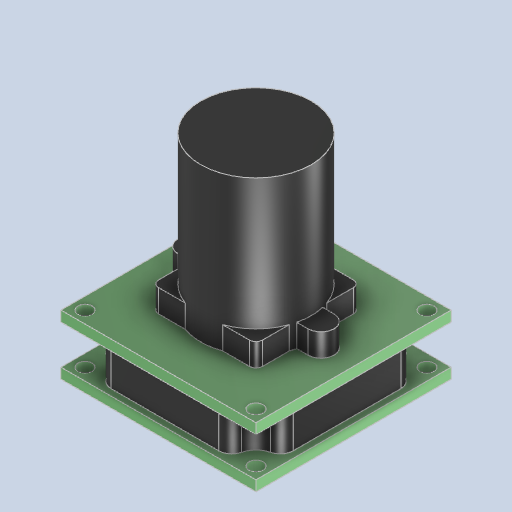
# Autodesk Inventor part: e-CAM50_CUNX
Saved by Autodesk Inventor 2022.3 (Build 263350000, 350)
## iProperties
Created: 2023-04-07
Part Number: e-CAM50_CUNX
Material: Generic
Document SubType Name: Modeling
Designer: Masato Kubotera
Density: 1 g/cm^3
Appearance: 光沢 - 黒
Catalog Web Link: https://www.e-consystems.com/nvidia-cameras/jetson-nx-cameras/5mp-mipi-camera-board-jp.asp
Description: ReadyMade
Author: Masato Kubotera
Autodesk Inventor part; units mm, degrees
ref_plane "YZ Plane" through (0, 0, 0) normal (1, 0, 0) x (0, 1, 0)
ref_plane "XZ Plane" through (0, 0, 0) normal (0, 1, 0) x (-1, 0, 0)
sketch "スケッチ1" plane through (0, 0, 0) normal (0, 0, 1) x (1, 0, 0)
  line L0 (-15, -15) -> (15, -15)
  line L1 (15, -15) -> (15, 15)
  line L2 (15, 15) -> (-15, 15)
  line L3 (-15, 15) -> (-15, -15)
  line L4 (-15, -15) -> (15, 15) construction
  line L5 (15, -15) -> (-15, 15) construction
  line L6 (-15, 0) -> (15, 0) construction
  line L7 (0, 15) -> (0, -15) construction
  line L8 (-13.14, 13.14) -> (13.14, 13.14) construction
  line L9 (13.14, 13.14) -> (13.14, -13.14) construction
  line L10 (13.14, -13.14) -> (-13.14, -13.14) construction
  line L11 (-13.14, -13.14) -> (-13.14, 13.14) construction
  line L12 (-13.14, 13.14) -> (13.14, -13.14) construction
  line L13 (13.14, 13.14) -> (-13.14, -13.14) construction
  circle A0 centre (0, 0) radius 8.5
  line L14 (-7, 8) -> (7, 8)
  line L15 (8, 7) -> (8, -7)
  line L16 (7, -8) -> (-7, -8)
  line L17 (-8, -7) -> (-8, 7)
  line L18 (-8, 8) -> (8, -8) construction
  line L19 (8, 8) -> (-8, -8) construction
  arc A1 (-8, -7) -> (-7, -8) centre (-7, -7) ccw
  arc A2 (7, -8) -> (8, -7) centre (7, -7) ccw
  arc A3 (8, 7) -> (7, 8) centre (7, 7) ccw
  arc A4 (-7, 8) -> (-8, 7) centre (-7, 7) ccw
  arc A5 (-2, -10) -> (2, -10) centre (0, -10) ccw
  line L20 (-2, -10) -> (-2, -8)
  line L21 (2, -10) -> (2, -8)
  arc A6 (2, 10) -> (-2, 10) centre (0, 10) ccw
  line L22 (-2, 10) -> (-2, 8)
  line L23 (2, 10) -> (2, 8)
  circle A7 centre (-13.14, -13.14) radius 1.1
  circle A8 centre (13.14, -13.14) radius 1.1
  circle A9 centre (-13.14, 13.14) radius 1.1
  circle A10 centre (13.14, 13.14) radius 1.1
  circle A11 centre (-13.14, -13.14) radius 2 construction
  circle A12 centre (13.14, -13.14) radius 2 construction
  circle A13 centre (-13.14, 13.14) radius 2 construction
  circle A14 centre (13.14, 13.14) radius 2 construction
  arc A15 (-10.219, -12.456) -> (-12.456, -10.219) centre (-13.14, -13.14) ccw
  line L24 (-14, -8.2717) -> (-14, 8.2717)
  line L25 (-8.2717, -14) -> (8.2717, -14)
  arc A16 (-14, -8.2717) -> (-12.456, -10.219) centre (-12, -8.2717) ccw
  arc A17 (-10.219, -12.456) -> (-8.2717, -14) centre (-8.2717, -12) ccw
  arc A18 (-12.456, 10.219) -> (-10.219, 12.456) centre (-13.14, 13.14) ccw
  line L26 (-8.2717, 14) -> (8.2717, 14)
  arc A19 (-12.456, 10.219) -> (-14, 8.2717) centre (-12, 8.2717) ccw
  arc A20 (-8.2717, 14) -> (-10.219, 12.456) centre (-8.2717, 12) ccw
  arc A21 (12.456, -10.219) -> (10.219, -12.456) centre (13.14, -13.14) ccw
  line L27 (14, -8.2717) -> (14, 8.2717)
  arc A22 (12.456, -10.219) -> (14, -8.2717) centre (12, -8.2717) ccw
  arc A23 (8.2717, -14) -> (10.219, -12.456) centre (8.2717, -12) ccw
  arc A24 (14, 8.2717) -> (12.456, 10.219) centre (12, 8.2717) ccw
  arc A25 (10.219, 12.456) -> (12.456, 10.219) centre (13.14, 13.14) ccw
  arc A26 (10.219, 12.456) -> (8.2717, 14) centre (8.2717, 12) ccw
  point P0 (-10.2659, -14)
  point P1 (-14, -10.2659)
  point P2 (-8, -2.8723)
  point P3 (-8, 2.8723)
  point P4 (-2.8723, 8)
  point P5 (-2, 8.2614)
  point P6 (2, 8.2614)
  point P7 (2.8723, 8)
  point P8 (8, 2.8723)
  point P9 (8, -2.8723)
  point P10 (2.8723, -8)
  point P11 (2, -8.2614)
  point P12 (-2, -8.2614)
  point P13 (-2.8723, -8)
  dimension "d0" = 30
  dimension "d1" = 30
  dimension "d2" = 26.28
  dimension "d3" = 26.28
  dimension "d4" = 17
  dimension "d5" = 16
  dimension "d6" = 16
  dimension "d7" = 1
  dimension "d8" = 20
  dimension "d9" = 2
  dimension "d10" = 2.2
  dimension "d11" = 4
  dimension "d12" = 2
  dimension "d13" = 3
  dimension "d14" = 1
  dimension "d15" = 1
  constraints: 56 end point, 38 point on circle, 36 symmetric about line, 27 centre point, 13 tangent, 12 point on line, 10 midpoint, 8 parallel, 4 coincident, 4 equal radius, 4 perpendicular, 3 horizontal, 16 other
  measures "d0" distance of L2.end L1.end
  measures "d1" distance of L1.end L0.end
  measures "d2" distance of L9.end L10.end
  measures "d3" distance of L8.end L9.end
  measures "d4" diameter of A0
  measures "d5" distance of L18.end L19.end
  measures "d6" distance of L19.start L18.end
  measures "d7" radius of A1
  measures "d8" distance of A6.centre A5.centre
  measures "d9" radius of A5
  measures "d10" diameter of A7
  measures "d11" diameter of A11
  measures "d12" radius of A16
  measures "d13" radius of A15
  measures "d14" distance between parallel lines of L0 L25
  measures "d15" distance between parallel lines of L3 L24
extrude "押し出し1" add sketch "スケッチ1" along normal blind 9.2 contours L3 L2 L1 L0 | A15 A16 L24 A19 A18 A20 L26 A26 A25 A24 L27 A22 A21 A23 L25 A17
extrude "押し出し2" cut sketch "スケッチ1" along normal blind 7.6 contours L3 L2 L1 L0
extrude "押し出し3" add sketch "スケッチ1" along normal blind 1.6 contours L3 L2 L1 L0
extrude "押し出し4" add sketch "スケッチ1" along normal blind 12.7 contours A0 L14 A3 L15 | L15 A2 L16 A0 | A0 L22 A6 L23 | L21 A5 L20 A0 | A0 L17 A4 L14 | L16 A1 L17 A0
extrude "押し出し5" add sketch "スケッチ1" along normal blind 32.8 contours A0 L15 | L15 A0 L16 L17 L14 | L14 L23 A0 | A0 L21 L16 | L23 L14 L22 A0 | A0 L20 L16 L21 | L22 L14 A0 | A0 L16 L20 | L17 A0
ref_plane "作業平面1" through (0, 0, 27.5) normal (0, 0, 1) x (1, 0, 0)
sketch "focus of the lens" plane through (0, 0, 27.5) normal (0, 0, 1) x (1, 0, 0)
  point P0 (0, 0)
  point P1 (0, 0)
  constraints: 1 coincident
equation "\"d1\" = d0"
equation "\"d3\" = d2"
equation "\"d6\" = d5"
equation "\"d15\" = d14"
